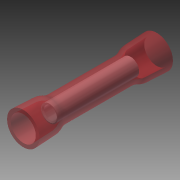
# Autodesk Inventor part: 22-18 double sided female tube heat shrink red
Saved by Autodesk Inventor 2014 (Build 180170000, 170)
## iProperties
Created: 2013-07-20
Part Number: 22-18 double sided female tube heat shrink red
Material: Generic
Document SubType Name: Modeling
Designer: Saville
Mass: 0.268121 g
Surface Area: 9.39649 cm^2
Volume: 0.268121 cm^3
Density: 1 g/cm^3
Appearance: Default
Author: Saville
Autodesk Inventor part; units mm, degrees
ref_plane "YZ Plane" through (0, 0, 0) normal (1, 0, 0) x (0, 1, 0)
ref_plane "XZ Plane" through (0, 0, 0) normal (0, 1, 0) x (-1, 0, 0)
ref_plane "XY Plane" through (0, 0, 0) normal (0, 0, 1) x (1, 0, 0)
sketch "Sketch1" plane through (0, 0, 0) normal (0, 0, 1) x (1, 0, 0)
  circle A0 centre (0, 0) radius 2.2225
  dimension "d0" = 4.445
  constraints: 1 centre point, 1 coincident
  measures "d0" diameter of A0
extrude "Extrusion1" add sketch "Sketch1" along normal mid plane 13.8176
sketch "Sketch4" plane through (0, 0, 6.9088) normal (0, 0, 1) x (1, 0, 0)
  circle A0 centre (0, 0) radius 2.7305
  dimension "d16" = 5.461
  constraints: 1 centre point, 1 coincident
  measures "d16" diameter of A0
extrude "Extrusion3" add sketch "Sketch4" along normal blind 5.2578 draft 2.5
fillet "Fillet3" radius 2.54 2 edges at (-2.7305, 0, 6.9088) (-2.2225, 0, 6.9088)
mirror "Mirror2" about plane through (0, 0, 0) normal (0, 0, 1) of "Extrusion3", "Fillet3"
shell "Shell1" thickness 0.6731 removed faces 2 at (-0.7385, 0.6543, 12.1666) at (-0.7385, 0.6543, -12.1666)
sketch "Sketch3" plane through (0, 0, 0) normal (1, 0, 0) x (0, 1, 0)
  line L0 (-1.5494, -7.4105) -> (-1.1811, -7.4105)
  line L1 (-1.1811, -7.4105) -> (-1.1811, 7.4105)
  line L2 (-1.1811, 7.4105) -> (-1.5494, 7.4105)
  line L3 (-1.5494, 7.4105) -> (-1.5494, -7.4105)
  line L4 (0, -17.3088) -> (0, 17.3088) projected
  arc A0 (-2.5104, -7.3447) -> (-2.2225, -6.17) centre (-4.7625, -6.17) ccw projected
  line L5 (-2.2225, -6.17) -> (-2.2225, 6.17) projected
  arc A1 (-2.2225, 6.17) -> (-2.5104, 7.3447) centre (-4.7625, 6.17) ccw projected
  arc A2 (-2.796, 8.4086) -> (-2.5104, 7.3447) centre (-0.2584, 8.5194) ccw projected
  line L6 (-2.796, 8.4086) -> (-2.9601, 12.1666) projected
  line L7 (-2.9601, 12.1666) -> (-2.2863, 12.1666) projected
  line L8 (-2.2863, 12.1666) -> (-2.1235, 8.4379) projected
  arc A3 (-2.1235, 8.4379) -> (-1.9137, 7.656) centre (-0.2584, 8.5194) ccw projected
  arc A4 (-1.5494, 6.17) -> (-1.9137, 7.656) centre (-4.7625, 6.17) ccw projected
  line L9 (-1.5494, 6.17) -> (-1.5494, -6.17) projected
  arc A5 (-1.9137, -7.656) -> (-1.5494, -6.17) centre (-4.7625, -6.17) ccw projected
  arc A6 (-1.9137, -7.656) -> (-2.1235, -8.4379) centre (-0.2584, -8.5194) ccw projected
  line L10 (-2.1235, -8.4379) -> (-2.2863, -12.1666) projected
  line L11 (-2.2863, -12.1666) -> (-2.9601, -12.1666) projected
  line L12 (-2.9601, -12.1666) -> (-2.796, -8.4086) projected
  arc A7 (-2.5104, -7.3447) -> (-2.796, -8.4086) centre (-0.2584, -8.5194) ccw projected
  arc A8 (2.2225, -6.17) -> (2.5104, -7.3447) centre (4.7625, -6.17) ccw projected
  arc A9 (2.796, -8.4086) -> (2.5104, -7.3447) centre (0.2584, -8.5194) ccw projected
  line L13 (2.796, -8.4086) -> (2.9601, -12.1666) projected
  line L14 (2.9601, -12.1666) -> (2.2863, -12.1666) projected
  line L15 (2.2863, -12.1666) -> (2.1235, -8.4379) projected
  arc A10 (2.1235, -8.4379) -> (1.9137, -7.656) centre (0.2584, -8.5194) ccw projected
  arc A11 (1.5494, -6.17) -> (1.9137, -7.656) centre (4.7625, -6.17) ccw projected
  line L16 (1.5494, -6.17) -> (1.5494, 6.17) projected
  arc A12 (1.9137, 7.656) -> (1.5494, 6.17) centre (4.7625, 6.17) ccw projected
  arc A13 (1.9137, 7.656) -> (2.1235, 8.4379) centre (0.2584, 8.5194) ccw projected
  line L17 (2.1235, 8.4379) -> (2.2863, 12.1666) projected
  line L18 (2.2863, 12.1666) -> (2.9601, 12.1666) projected
  line L19 (2.9601, 12.1666) -> (2.796, 8.4086) projected
  arc A14 (2.5104, 7.3447) -> (2.796, 8.4086) centre (0.2584, 8.5194) ccw projected
  arc A15 (2.5104, 7.3447) -> (2.2225, 6.17) centre (4.7625, 6.17) ccw projected
  line L20 (2.2225, 6.17) -> (2.2225, -6.17) projected
  point P0 (0, 0)
  point P1 (-1.5494, 6.6485)
  point P2 (-1.5494, -6.6485)
  dimension "d9" = 0.3683
  constraints: 8 end point, 2 parallel, 1 horizontal, 1 perpendicular
  measures "d9" distance between parallel lines of L1 L3
revolve "Revolution1" add sketch "Sketch3" angle 360 about axis through (0, 0, -10) along (0, 0, 1) separate body contours L3 L2 L1 L0
chamfer "Chamfer1" distance 0.2032 angle 45 2 edges at (0, 1.1811, 7.4105) (0, 1.1811, -7.4105)
body "Solid1"
body "Solid2"
